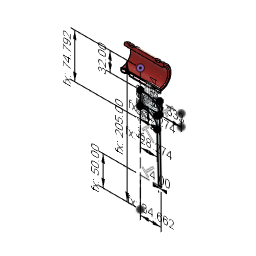
bike adapter conico v16 (Autodesk Fusion 360 design; units mm, degrees)
Autodesk Fusion 360 part; units mm, degrees
sketch "Sketch1" plane through (0, 0, 0) normal (1, 0, 0) x (0, 1, 0)
  circle A0 centre (0, 0) radius 15 construction
  circle A1 centre (0, 0) radius 20 construction
  line L0 (0, 0) -> (6.8404, 18.7939) construction
  line L1 (0, 0) -> (20, 0) construction
  line L2 (0, 2.5) -> (0, 20) construction
  line L3 (0, 0) -> (-6.8404, 18.7939) construction
  arc A2 (-5.1303, 14.0954) -> (5.1303, 14.0954) centre (0, 0) ccw
  line L4 (-6.8404, 18.7939) -> (-5.1303, 14.0954)
  line L5 (6.8404, 18.7939) -> (5.1303, 14.0954)
  arc A3 (-6.8404, 18.7939) -> (6.8404, 18.7939) centre (0, 0) ccw
  dimension "handlebar_dia" = 30
  dimension "d3" = 5
  dimension "d4" = 70
  constraint coincident A0.centre A1.centre
  constraint horizontal L1
  constraint symmetric A0.centre L2 A1.centre
  constraint symmetric L0.end L2 L3.end
  constraint coincident A0 A2.end
  constraint coincident L0 A2.end
  constraint parallel L3 L4
  constraint coincident A1 L0.end
  constraint coincident L0 L5.start
  measures "handlebar_dia" diameter of A0
  measures "d4" angle of L0 L1
extrude "Extrude1" add sketch "Sketch1" along normal blind 32.6624
sketch "Sketch2" plane through (0, 0, 0) normal (0, 1, 0) x (1, 0, 0)
  line L0 (0, -20) -> (0, 20)
  line L1 (18.6624, -20) -> (25.1624, -20)
  line L2 (25.1624, -20) -> (25.1624, -18)
  line L3 (25.1624, -18) -> (18.6624, -18)
  line L4 (18.6624, -18) -> (18.6624, -20)
  point P0 (0, -20)
  dimension "d10" = 6.5
  dimension "d11" = 2
  dimension "d170" = 18.6624
  constraint horizontal L1
  constraint vertical L2
  constraint horizontal L3
  constraint vertical L4
  measures "d10" distance of L1.start L1.end
  measures "d11" distance of L1.start L3.end
  measures "d170" distance of P0 L1.start
revolve "Revolve1" cut sketch "Sketch2" angle 360 about axis through (1.75, 0, 0) along (1, 0, 0)
fillet "Fillet1" radius 1.5 1 edges at (32.6624, 0, -15)
fillet "Fillet6" radius 1.5 3 edges at (18.6624, 0, -20) (25.1624, 0, -20) (32.6624, 0, -20)
mirror "Mirror1" about plane through (0, 0, 0) normal (1, 0, 0) of bodies 1 merged
sketch "Sketch10" plane through (0, 0, 0) normal (0, 1, 0) x (1, 0, 0)
  line L0 (0, 0) -> (0, 205) construction
  line L1 (0, 32) -> (68.3333, 32) construction
  line L2 (0, 51.3643) -> (68.3333, 51.3643) construction
  line L3 (32.2739, 32) -> (32.2739, 51.3643) construction
  line L4 (0, 32) -> (32.2739, 32)
  line L5 (32.2739, 32) -> (32.2739, 51.3643)
  spline S0 degree 2 poles (0, 32) (32.2739, 32) (32.2739, 51.3643) knots 0 0 0 1 1 1
  line L6 (0, 74.7917) -> (28.2739, 74.7917) construction
  line L7 (0, 55) -> (28.2739, 55) construction
  line L8 (0, 55) -> (28.2739, 55)
  line L9 (28.2739, 55) -> (28.2739, 74.7917)
  spline S1 degree 2 poles (0, 55) (28.2739, 55) (28.2739, 74.7917) knots 0 0 0 1 1 1
  line L10 (0, 155) -> (34.6624, 155) construction
  line L11 (32.2739, 51.3643) -> (34.6624, 155)
  line L12 (34.6624, 155) -> (30.6624, 155)
  line L13 (30.6624, 155) -> (28.2739, 74.7917)
  line L14 (0, 32) -> (0, 55)
  dimension "d83" = 205
  dimension "d84" = 68.3333
  dimension "d85" = 32
  dimension "d88" = -19.3643
  dimension "d89" = 32.2739
  dimension "d91" = 28.2739
  dimension "d92" = 74.7917
  dimension "d93" = 19.7917
  dimension "d94" = 34.6624
  dimension "d96" = 50
  dimension "d98" = 4
  constraint coincident L0.start origin
  constraint vertical L0
  constraint coincident L0 L1.start
  constraint perpendicular L0 L1
  constraint coincident L1 L3.start
  constraint coincident L2 L3.end
  constraint perpendicular L2 L3
  constraint coincident L3.start L4.end
  constraint coincident L0 L6.start
  constraint perpendicular L0 L6
  constraint coincident L7.end L8.end
  constraint coincident L0 L10.start
  constraint perpendicular L0 L10
  constraint coincident L10 L12.end
  constraint perpendicular L7 L14
  measures "d83" distance of L0.start L0.end
  measures "d84" distance of L1.start L1.end
  measures "d85" distance of L0.start L1.start
  measures "d89" distance of L2.start L3.end
  measures "d91" distance of L6.start L6.end
  measures "d92" distance of L0.start L6.start
  measures "d94" distance of L10.start L10.end
  measures "d96" distance of L0.end L10.start
  measures "d98" distance of L10.end L12.end
revolve "Revolve4" [rolled back] along angle 360
chamfer "Chamfer2" [rolled back] distance 2
fillet "Fillet12" [rolled back] radius 20
sketch "Sketch11" plane through (0, 0, 0) normal (0, 1, 0) x (1, 0, 0)
  circle A0 centre (0, 146) radius 4.5
  line L0 (-34.6624, 155) -> (34.6624, 155) construction
  dimension "d100" = 9
  dimension "d182" = 9
  measures "d100" diameter of A0
  measures "d182" distance of A0.centre L0
extrude "Extrude6" [rolled back] along distance 57.3248 taper angle 0
pattern_circular "C-Pattern3" [rolled back] total angle 180
pattern_linear "R-Pattern3" [rolled back] u space distance 20 v space distance 0
ref_plane "WorkPlane3" through (0, 0, -25) normal (0, 0, 1) x (1, 0, 0)
sketch "Sketch12" plane through (0, 0, -25) normal (0, 0, 1) x (1, 0, 0)
  ellipse E0 centre (0, 0) end of major axis (0, -16) minor radius 13.5
  line L0 (0, 16) -> (0, -16)
  line L1 (-13.5, 0) -> (13.5, 0)
  dimension "d171" = 32
  dimension "d172" = 27
  constraint coincident E0.centre origin
  constraint vertical L0
  constraint coincident E0 L0.start
  constraint coincident E0 L0.end
  constraint coincident E0 L1.start
  constraint coincident E0 L1.end
  measures "d171" distance of E0
extrude "Extrude7" [rolled back] side1offset 0 taper angle 0 side2offset 0 side2taper angle 0
fillet "Fillet4" [rolled back] radius 11.2739 radius 7.5
ref_plane "WorkPlane4" through (0, 0, -25) normal (0, 0, 1) x (1, 0, 0)
sketch "Sketch13" plane through (0, 0, -25) normal (0, 0, 1) x (1, 0, 0)
  line L0 (27.2739, 1.5) -> (31.2739, 1.5)
  line L1 (31.2739, 1.5) -> (31.2739, -1.5)
  line L2 (31.2739, -1.5) -> (27.2739, -1.5)
  line L3 (27.2739, -1.5) -> (27.2739, 1.5)
  line L4 (1.75, 0) -> (22.5, 0)
  dimension "d122" = 3
  dimension "d138" = 4
  dimension "d139" = 27.2739
  constraint horizontal L0
  constraint vertical L1
  constraint horizontal L2
  constraint vertical L3
  constraint symmetric L0 L2 L4
  measures "d122" distance of L0.start L2.end
  measures "d138" distance of L0.start L0.end
  measures "d139" distance of L3 origin
extrude "Extrude8" [rolled back] side1offset 0 taper angle 0 side2taper angle 0 against distance 20
mirror "Mirror6" [rolled back] mirror stitch tolerance 0.1
combine "Combine2" [rolled back]
equation "handlebar_dia = E_handle_dia"
equation "d5 = D_root_circ / 6.28 + 4 mm"
equation "d15 = E_handle_dia / 20"
equation "A_lng_unaff = 205 mm" comment "Unaffected arm length"
equation "B_lng_affect = 130 mm" comment "Affected arm length"
equation "C_tip_circ = 165 mm" comment "Affected tip circumference"
equation "D_root_circ = 180 mm" comment "Affected root circumference"
equation "d83 = A_lng_unaff"
equation "d84 = A_lng_unaff / 3"
equation "tip_dia_ext = C_tip_circ / 3.14 + 12 mm" comment "External tip diameter"
equation "root_dia_ext = D_root_circ / 3.14 + 12 mm" comment "External root diameter"
equation "d88 = -tip_dia_ext / 2 * 0.6"
equation "d89 = tip_dia_ext / 2"
equation "miss_arm_lenght = A_lng_unaff - B_lng_affect - 20 mm"
equation "d91 = d89 - 4 mm"
equation "d92 = miss_arm_lenght + d93"
equation "d93 = d91 * 0.7"
equation "d94 = root_dia_ext / 2"
equation "d96 = B_lng_affect - F_lng_affect_inner_elbow"
equation "d100 = D_root_circ * 0.05"
equation "d102 = D_root_circ / 3.14"
equation "vent_hole_no = 4" comment "Number of venting holes"
equation "d107 = vent_hole_no"
equation "d121 = -E_handle_dia / 2 - 10 mm"
equation "E_handle_dia = 30 mm" comment "Handlebar diameter"
equation "d139 = C_tip_circ / 6.28 + 1 mm"
equation "d141 = E_handle_dia / 20"
equation "F_lng_affect_inner_elbow = 80 mm"
equation "avg_circ = ( C_tip_circ + D_root_circ ) / 2"
equation "d170 = D_root_circ / 6.28 - 10 mm"
equation "d171 = E_handle_dia + 2 mm"
equation "d172 = E_handle_dia - 3 mm"
equation "d174 = C_tip_circ / 6.28 - 15 mm"
equation "d178 = E_handle_dia / 4"
named bodies: "bike_adapt"
